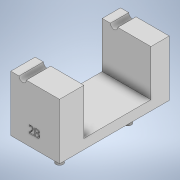
# Autodesk Inventor part: Support_2B
Saved by Autodesk Inventor 2021 (Build 250183000, 183)
## iProperties
Created: 2021-04-14
Part Number: Support_2B
Material: Generic
Document SubType Name: Modeling
Designer: Jawal
Density: 1 g/cm^3
Appearance: Default
Author: Jawal
Autodesk Inventor part; units mm, degrees
note: some values were not read from the file. Chosen so that the rebuilt part matches the saved one: direction of "Emboss1".
ref_plane "YZ Plane" through (0, 0, 0) normal (1, 0, 0) x (0, 1, 0)
ref_plane "XZ Plane" through (0, 0, 0) normal (0, 1, 0) x (-1, 0, 0)
ref_plane "XY Plane" through (0, 0, 0) normal (0, 0, 1) x (1, 0, 0)
sketch "Sketch1" plane through (0, 0, 0) normal (1, 0, 0) x (0, 1, 0)
  line L0 (11.4385, 17.5) -> (-11.4385, 17.5)
  line L1 (-11.4385, 17.5) -> (-11.4385, -27.5)
  line L2 (-11.4385, -27.5) -> (11.4385, -27.5)
  line L3 (11.4385, -27.5) -> (11.4385, 17.5)
  point P0 (0, 0)
  dimension "d0" = 45
  dimension "d1" = 22.877
  dimension "d2" = 11.4385
  dimension "d15" = 17.5
  constraints: 8 end point, 2 parallel, 1 horizontal, 1 perpendicular
  measures "d0" distance of L2.end L0.start
  measures "d1" distance of L1.end L2.end
  measures "d2" distance from line of point (0, 0) L3
  measures "d15" distance from line of L0 point (0, 0)
extrude "Extrusion1" add sketch "Sketch1" along normal blind 20
sketch "Sketch2" plane through (0, -11.4385, -27.5) normal (0, -1, 0) x (1, 0, 0)
  circle A0 centre (16.5, 41.5) radius 1.5
  circle A1 centre (16.5, 13.5) radius 1.5
  line L0 (0, 0) -> (20, 0) projected
  line L1 (0, 45) -> (20, 45) projected
  line L2 (20, 0) -> (20, 45) projected
  point P0 (0, 27.5)
  dimension "d6" = 3
  dimension "d7" = 3
  dimension "d8" = 28
  dimension "d10" = 3.5
  dimension "d12" = 3.5
  constraints: 2 centre point
  measures "d6" diameter of A0
  measures "d7" diameter of A1
  measures "d8" distance of A1.centre A0.centre
  measures "d10" distance from line of L1 A0.centre
  measures "d12" distance from line of L2 A0.centre
extrude "Extrusion2" add sketch "Sketch2" along normal blind 3
sketch "Sketch3" plane through (20, 0, 0) normal (1, 0, 0) x (0, 0, -1)
  line L0 (27.5, 11.4385) -> (-17.5, 11.4385) projected
  line L1 (-7.5, 11.4385) -> (20, 11.4385)
  line L2 (20, 11.4385) -> (20, -7.4385)
  line L3 (20, -7.4385) -> (-7.5, -7.4385)
  line L4 (-7.5, -7.4385) -> (-7.5, 11.4385)
  line L5 (27.5, -11.4385) -> (27.5, 11.4385) projected
  line L6 (-17.5, -11.4385) -> (27.5, -11.4385) projected
  line L7 (-17.5, 11.4385) -> (-17.5, -11.4385) projected
  point P0 (0, 0)
  dimension "d17" = 7.5
  dimension "d18" = 4
  dimension "d25" = 10
  constraints: 8 end point, 2 parallel, 1 horizontal, 1 perpendicular, 1 point on line
  measures "d17" distance between parallel lines of L2 L5
  measures "d18" distance between parallel lines of L6 L3
  measures "d25" distance between parallel lines of L7 L4
extrude "Extrusion3" cut sketch "Sketch3" against normal through all contours L2 L3 L4 L0
sketch "Sketch4" plane through (0, -11.4385, -27.5) normal (0, 0, -1) x (-1, 0, 0)
  line L0 (0, 22.877) -> (-20, 22.877) projected
  arc A0 (-6.387, 22.877) -> (-3.387, 22.877) centre (-4.887, 22.877) ccw
  line L1 (-20, 0) -> (-20, 22.877) projected
  point P0 (0, 11.4385)
  dimension "d21" = 3
  dimension "d22" = 15.113
  constraints: 3 point on line, 2 point on circle, 1 centre point
  measures "d21" diameter of A0
  measures "d22" distance from line of L1 A0.centre
extrude "Extrusion4" cut sketch "Sketch4" against normal through all
sketch "Sketch5" plane through (0, -11.4385, 17.5) normal (0, 0, 1) x (1, 0, 0)
  line L0 (7.2589, 7.7565) -> (13.3951, 7.7565) construction
  line L1 (13.3951, 7.7565) -> (13.3951, 2.3021) construction
  line L2 (13.3951, 2.3021) -> (7.2589, 2.3021) construction
  line L3 (7.2589, 2.3021) -> (7.2589, 7.7565) construction
  line L4 (9.3609, 4.6443) -> (7.4812, 4.6443)
  line L5 (7.4812, 4.6443) -> (7.4812, 5.0765)
  spline S0 degree 2 poles (7.4812, 5.0765) (7.6837, 5.2667) (8.0444, 5.6199) (8.2173, 5.8101) knots 0 0 0 1 2 2 2
  spline S1 degree 2 poles (8.2173, 5.8101) (8.5655, 6.193) (8.82, 6.6524) (8.82, 6.8969) knots 0 0 0 1 2 2 2
  spline S2 degree 2 poles (8.82, 6.8969) (8.82, 7.0254) (8.7409, 7.218) (8.6693, 7.2798) knots 0 0 0 1 2 2 2
  spline S3 degree 2 poles (8.6693, 7.2798) (8.5977, 7.3415) (8.4099, 7.4033) (8.2963, 7.4033) knots 0 0 0 1 2 2 2
  spline S4 degree 2 poles (8.2963, 7.4033) (8.1876, 7.4033) (7.9653, 7.3489) (7.8641, 7.307) knots 0 0 0 1 2 2 2
  spline S5 degree 2 poles (7.8641, 7.307) (7.7776, 7.2724) (7.6171, 7.1736) (7.5677, 7.139) knots 0 0 0 1 2 2 2
  line L6 (7.5677, 7.139) -> (7.5454, 7.139)
  line L7 (7.5454, 7.139) -> (7.5454, 7.5737)
  spline S6 degree 2 poles (7.5454, 7.5737) (7.6714, 7.6355) (8.1234, 7.7565) (8.326, 7.7565) knots 0 0 0 1 2 2 2
  spline S7 degree 2 poles (8.326, 7.7565) (8.7533, 7.7565) (9.2349, 7.3045) (9.2349, 6.9192) knots 0 0 0 1 2 2 2
  spline S8 degree 2 poles (9.2349, 6.9192) (9.2349, 6.7389) (9.1509, 6.4375) (9.0768, 6.3091) knots 0 0 0 1 2 2 2
  spline S9 degree 2 poles (9.0768, 6.3091) (9.0027, 6.1757) (8.7878, 5.9139) (8.6693, 5.7879) knots 0 0 0 1 2 2 2
  spline S10 degree 2 poles (8.6693, 5.7879) (8.4766, 5.5779) (8.0048, 5.1284) (7.8641, 4.9975) knots 0 0 0 1 2 2 2
  line L8 (7.8641, 4.9975) -> (9.3609, 4.9975)
  line L9 (9.3609, 4.9975) -> (9.3609, 4.6443)
  spline S11 degree 2 poles (11.9223, 5.5804) (11.9223, 5.3532) (11.7494, 5.0049) (11.6061, 4.8913) knots 0 0 0 1 2 2 2
  spline S12 degree 2 poles (11.6061, 4.8913) (11.4332, 4.7579) (11.0405, 4.6443) (10.7293, 4.6443) knots 0 0 0 1 2 2 2
  line L10 (10.7293, 4.6443) -> (9.8549, 4.6443)
  line L11 (9.8549, 4.6443) -> (9.8549, 7.6923)
  line L12 (9.8549, 7.6923) -> (10.6626, 7.6923)
  spline S13 degree 2 poles (10.6626, 7.6923) (10.9886, 7.6923) (11.3147, 7.6503) (11.4629, 7.5688) knots 0 0 0 1 2 2 2
  spline S14 degree 2 poles (11.4629, 7.5688) (11.6284, 7.4823) (11.779, 7.1983) (11.779, 7.0056) knots 0 0 0 1 2 2 2
  spline S15 degree 2 poles (11.779, 7.0056) (11.779, 6.7907) (11.5518, 6.4499) (11.3517, 6.3535) knots 0 0 0 1 2 2 2
  line L13 (11.3517, 6.3535) -> (11.3517, 6.3387)
  spline S16 degree 2 poles (11.3517, 6.3387) (11.6234, 6.2646) (11.9223, 5.8719) (11.9223, 5.5804) knots 0 0 0 1 2 2 2
  spline S17 degree 2 poles (11.4999, 5.5631) (11.4999, 5.736) (11.4011, 5.9583) (11.2529, 6.0374) knots 0 0 0 1 2 2 2
  spline S18 degree 2 poles (11.2529, 6.0374) (11.1566, 6.0868) (10.9293, 6.1164) (10.7194, 6.1164) knots 0 0 0 1 2 2 2
  line L14 (10.7194, 6.1164) -> (10.26, 6.1164)
  line L15 (10.26, 6.1164) -> (10.26, 4.9901)
  line L16 (10.26, 4.9901) -> (10.5885, 4.9901)
  spline S19 degree 2 poles (10.5885, 4.9901) (10.8552, 4.9901) (11.1615, 5.0395) (11.2801, 5.1185) knots 0 0 0 1 2 2 2
  spline S20 degree 2 poles (11.2801, 5.1185) (11.3937, 5.2) (11.4999, 5.4026) (11.4999, 5.5631) knots 0 0 0 1 2 2 2
  spline S21 degree 2 poles (11.3567, 6.9488) (11.3567, 7.0575) (11.2826, 7.2205) (11.201, 7.2674) knots 0 0 0 1 2 2 2
  spline S22 degree 2 poles (11.201, 7.2674) (11.1022, 7.3218) (10.8627, 7.3465) (10.6478, 7.3465) knots 0 0 0 1 2 2 2
  line L17 (10.6478, 7.3465) -> (10.26, 7.3465)
  line L18 (10.26, 7.3465) -> (10.26, 6.4548)
  line L19 (10.26, 6.4548) -> (10.7194, 6.4548)
  spline S23 degree 2 poles (10.7194, 6.4548) (10.9096, 6.4548) (11.0899, 6.4943) (11.1862, 6.5561) knots 0 0 0 1 2 2 2
  spline S24 degree 2 poles (11.1862, 6.5561) (11.2801, 6.6154) (11.3567, 6.8055) (11.3567, 6.9488) knots 0 0 0 1 2 2 2
  point P0 (0, 11.4385)
  constraints: 2 other
emboss "Emboss1" sketch "Sketch5" operation cut depth 1 direction (0, 0, -1)
equation "\"d2\" = 0.5 * d1"
body "Solid1"
